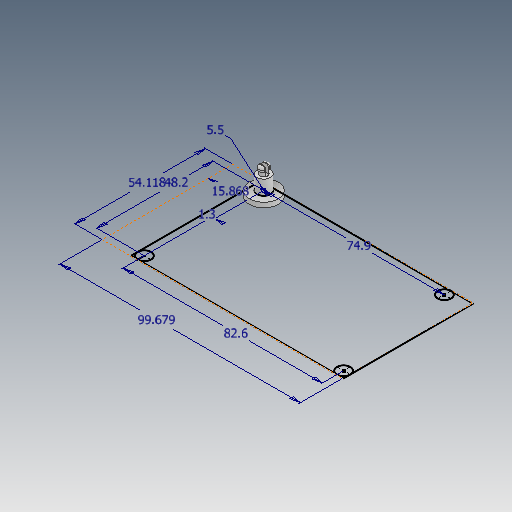
# Autodesk Inventor part: arduino_mega_standoffs_retention-clips_single
Saved by Autodesk Inventor 2025.1 (Build 291241000, 241)
## iProperties
Created: 2026-06-20
Part Number: arduino_mega_standoffs_retention-clips_single
Material: Generic
Document SubType Name: Modeling
Designer: Aiden
Density: 1 g/cm^3
Appearance: Default
Author: Aiden
Autodesk Inventor part; units mm, degrees
ref_plane "YZ Plane" through (0, 0, 0) normal (1, 0, 0) x (0, 1, 0)
ref_plane "XZ Plane" through (0, 0, 0) normal (0, 1, 0) x (-1, 0, 0)
ref_plane "XY Plane" through (0, 0, 0) normal (0, 0, 1) x (1, 0, 0)
sketch "Sketch1" plane through (0, 0, 0) normal (0, 1, 0) x (-1, 0, 0)
  circle A0 centre (43.0199, -7.0958) radius 2.75
  circle A1 centre (-31.8801, -7.0958) radius 2.75
  circle A2 centre (44.3199, 41.1042) radius 2.75
  circle A3 centre (-38.2801, 41.1042) radius 2.75
  line L0 (58.8879, -10.055) -> (-40.7911, -10.055) construction
  line L1 (-40.7911, -10.055) -> (-40.7911, 44.0634) construction
  line L2 (-40.7911, 44.0634) -> (58.8879, 44.0634) construction
  line L3 (58.8879, 44.0634) -> (58.8879, -10.055) construction
  line L4 (43.0199, -7.0958) -> (43.0199, -10.055)
  line L5 (44.3199, 41.1042) -> (44.3199, 44.0634)
  line L6 (47.0699, -9.8458) -> (-41.0301, -9.8458)
  line L7 (-41.0301, -9.8458) -> (-41.0301, 43.8542)
  line L8 (-41.0301, 43.8542) -> (47.0699, 43.8542)
  line L9 (47.0699, 43.8542) -> (47.0699, -9.8458)
  dimension "d0" = 5.5
  dimension "d1" = 74.9
  dimension "d2" = 1.3
  dimension "d3" = 48.2
  dimension "d5" = 82.6
  dimension "d9" = 15.868
  dimension "d10" = 54.1184
  dimension "d11" = 99.679
  constraints: 20 end point, 5 parallel, 4 centre point, 4 perpendicular, 4 tangent, 3 coincident, 3 equal radius, 2 horizontal, 2 horizontal alignment, 2 point on line
  measures "d0" diameter of A0
  measures "d1" distance of A1.centre L4.start
  measures "d2" horizontal distance of L5.start L4.start
  measures "d3" vertical distance of L4.start L5.start
  measures "d5" distance of A3.centre L5.start
  measures "d9" distance from line of L3 L4.start
  measures "d10" distance of L2.end L0.start
  measures "d11" distance of L1.end L2.end
extrude "Extrusion2" add sketch "Sketch1" along normal blind 6 contours A0
sketch "Sketch4" plane through (-43.0199, 6, -7.0958) normal (0, 1, 0) x (1, 0, 0)
  circle A0 centre (0, 0) radius 2.75 projected
  circle A1 centre (0, 0) radius 1.575
  point P0 (43.0199, -7.0958)
  dimension "d24" = 3.15
  constraints: 1 centre point, 1 coincident
  measures "d24" diameter of A1
extrude "Extrusion3" add sketch "Sketch4" along normal blind 1.8 contours A1
sketch "Sketch5" plane through (-43.0199, 7.8, -7.0958) normal (0, 1, 0) x (1, 0, 0)
  line L0 (-1.575, -0.575) -> (1.575, -0.575)
  line L1 (1.575, -0.575) -> (1.575, 0.575)
  line L2 (1.575, 0.575) -> (-1.575, 0.575)
  line L3 (-1.575, 0.575) -> (-1.575, -0.575)
  line L4 (-1.575, -0.575) -> (1.575, 0.575) construction
  line L5 (1.575, -0.575) -> (-1.575, 0.575) construction
  circle A0 centre (0, 0) radius 1.575 projected
  point P0 (43.0199, -7.0958)
  point P1 (-1.4663, -0.575)
  point P2 (1.4663, -0.575)
  point P3 (1.4663, 0.575)
  point P4 (-1.4663, 0.575)
  dimension "d27" = 1
  constraints: 12 end point, 2 midpoint, 2 parallel, 1 coincident, 1 horizontal, 1 perpendicular, 1 tangent
  measures "d27" distance edge to line of A0 L2
extrude "Extrusion4" cut sketch "Sketch5" against normal blind 6 contours A0 L2 L0
sketch "Sketch6" plane through (-43.0199, 7.8, -7.0958) normal (0, 1, 0) x (1, 0, 0)
  arc A0 (1.4663, 0.575) -> (-1.4663, 0.575) centre (0, 0) ccw construction
  line L0 (-1.4663, 0.575) -> (-1.4663, 0.975)
  line L1 (-1.4663, 0.575) -> (1.4663, 0.575) projected
  line L2 (1.4663, 0.575) -> (1.4663, 0.975)
  arc A1 (1.4663, 0.975) -> (-1.4663, 0.975) centre (0, 0.5477) ccw
  arc A2 (-1.4663, 0.575) -> (-1.4663, -0.575) centre (0, 0) ccw construction
  line L3 (-1.575, 0) -> (1.575, 0) construction
  arc A3 (1.4663, -0.575) -> (1.4663, 0.575) centre (0, 0) ccw construction
  line L4 (-1.4663, -0.575) -> (-1.4663, -0.975)
  line L5 (-1.4663, -0.575) -> (1.4663, -0.575)
  line L6 (1.4663, -0.575) -> (1.4663, -0.975)
  arc A4 (-1.4663, -0.975) -> (1.4663, -0.975) centre (0, -0.5477) ccw
  point P0 (43.0199, -7.0958)
  point P1 (0, 1.575)
  point P2 (0, 2.075)
  dimension "d30" = 0.4
  dimension "d31" = 0.4
  dimension "d32" = 0.5
  constraints: 12 end point, 8 point on circle, 3 symmetric about line, 2 centre point, 1 horizontal, 1 perpendicular, 1 vertical, 1 other
  measures "d30" distance of L0.start L0.end
  measures "d31" distance of L1.end L2.end
  measures "d32" distance of point (0, 1.575) point (0, 2.075)
extrude "Extrusion5" add sketch "Sketch6" along normal blind 1.75
fillet "Fillet1" radius 1 6 edges at (-44.4862, 9.55, -6.3208) (-41.5537, 9.55, -6.3208) (-43.0199, 9.55, -5.0208) (-41.5537, 9.55, -7.8708) (-44.4862, 9.55, -7.8708) (-43.0199, 9.55, -9.1708)
sketch "Sketch7" plane through (-43.0199, 1.8, -7.0958) normal (0, 1, 0) x (1, 0, 0)
  line L0 (1.4663, -0.575) -> (-1.4663, -0.575) projected
  arc A0 (1.4663, -0.575) -> (1.4663, 0.575) centre (0, 0) ccw projected
  line L1 (-1.4663, 0.575) -> (1.4663, 0.575) projected
  arc A1 (-1.4663, 0.575) -> (-1.4663, -0.575) centre (0, 0) ccw projected
  point P0 (43.0199, -7.0958)
extrude "Extrusion6" add sketch "Sketch7" along normal blind 4
fillet "Fillet2" radius 0.575 2 edges at (-43.0199, 5.8, -7.6708) (-43.0199, 5.8, -6.5208)
sketch "Sketch16" plane through (-43.0199, 0, -7.0958) normal (0, -1, 0) x (1, 0, 0)
  circle A0 centre (0, 0) radius 6
  point P0 (43.0199, 7.0958)
  dimension "d56" = 12
  constraints: 1 centre point
  measures "d56" diameter of A0
extrude "Extrusion9" add sketch "Sketch16" along normal blind 2
body "Solid2"
